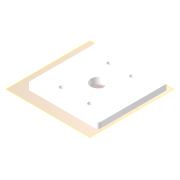
# Autodesk Inventor part: 20_Cube_Adapter_Zstage_manual
Saved by Autodesk Inventor 2022 (Build 260153000, 153)
## iProperties
Created: 2017-06-20
Part Number: 20_Cube_Adapter_Zstage_manual
Material: Generisch
Document SubType Name: Modeling
Designer: diederichbenedict
Density: 1 g/cm^3
Appearance: Weiß
Mass: 5.4697 g
Surface Area: 48.9743 cm^2
Volume: 5.4697 cm^3
Catalog Web Link: isInjectionmolded
Vendor: openUC2
d_part: 50,000 mm
d_o: 40,000 mm
d_i: 40,000 mm
Author: diederichbenedict
Autodesk Inventor part; units mm, degrees
ref_plane "YZ Plane" through (0, 0, 0) normal (1, 0, 0) x (0, 1, 0)
ref_plane "XZ Plane" through (0, 0, 0) normal (0, 1, 0) x (-1, 0, 0)
ref_plane "XY Plane" through (0, 0, 0) normal (0, 0, 1) x (1, 0, 0)
ref_plane "Arbeitsebene15" through (-38.58009, 58.540516, -23.010083) normal (0, 0, 1) x (1, 0, 0)
sketch "Skizze38" plane through (-38.58009, 58.540516, -23.010083) normal (0, 0, 1) x (1, 0, 0)
  circle A0 centre (27, 33.3) radius 3
  circle A1 centre (-8.3, 27) radius 3
  circle A2 centre (-2, -8.3) radius 3
  circle A3 centre (33.3, -2) radius 3
  circle A4 centre (27, -8.3) radius 3
  circle A5 centre (-8.3, -2) radius 3
  circle A6 centre (-2, 33.3) radius 3
  circle A7 centre (33.3, 27) radius 3
  line L0 (27.5, 29.5) -> (-2.5, 29.5)
  arc A8 (29.5, 27.5) -> (27.5, 29.5) centre (27.5, 27.5) ccw
  line L1 (29.5, 27.5) -> (29.5, -2.5)
  arc A9 (27.5, -4.5) -> (29.5, -2.5) centre (27.5, -2.5) ccw
  line L2 (-2.5, -4.5) -> (27.5, -4.5)
  arc A10 (-4.5, -2.5) -> (-2.5, -4.5) centre (-2.5, -2.5) ccw
  line L3 (-4.5, -2.5) -> (-4.5, 27.5)
  arc A11 (-2.5, 29.5) -> (-4.5, 27.5) centre (-2.5, 27.5) ccw
  circle A12 centre (33.5, 33.5) radius 2.5
  circle A13 centre (-8.5, -8.5) radius 2.5
  circle A14 centre (33.5, -8.5) radius 2.5
  circle A15 centre (-8.5, 33.5) radius 2.5
  line L4 (-11.75, -10.5) -> (-11.75, 8.25)
  arc A16 (-11.75, -10.5) -> (-10.5, -11.75) centre (-10.5, -10.5) ccw
  line L5 (8.25, -11.75) -> (-10.5, -11.75)
  line L6 (8.25, -13.877389) -> (8.25, -11.75)
  arc A17 (7.405556, -14.865216) -> (8.25, -13.877389) centre (7.25, -13.877389) ccw
  arc A18 (7.405556, -14.865216) -> (7.6, -17.35) centre (7.6, -16.1) ccw
  line L7 (17.4, -17.35) -> (7.6, -17.35)
  arc A19 (17.4, -17.35) -> (17.594444, -14.865216) centre (17.4, -16.1) ccw
  arc A20 (16.75, -13.877389) -> (17.594444, -14.865216) centre (17.75, -13.877389) ccw
  line L8 (16.75, -11.75) -> (16.75, -13.877389)
  line L9 (35.5, -11.75) -> (16.75, -11.75)
  arc A21 (35.5, -11.75) -> (36.75, -10.5) centre (35.5, -10.5) ccw
  line L10 (36.75, 6.487451) -> (36.75, -10.5)
  arc A22 (36.75, 6.487451) -> (36.55605, 6.521706) centre (36.65, 6.487451) ccw
  arc A23 (31.3, 7.45) -> (36.55605, 6.521706) centre (34.01, 7.45) ccw
  line L11 (31.3, 17.55) -> (31.3, 7.45)
  arc A24 (36.55605, 18.478294) -> (31.3, 17.55) centre (34.01, 17.55) ccw
  arc A25 (36.55605, 18.478294) -> (36.75, 18.512549) centre (36.65, 18.512549) ccw
  line L12 (36.75, 35.5) -> (36.75, 18.512549)
  arc A26 (36.75, 35.5) -> (35.5, 36.75) centre (35.5, 35.5) ccw
  line L13 (18.512549, 36.75) -> (35.5, 36.75)
  arc A27 (18.512549, 36.75) -> (18.478294, 36.55605) centre (18.512549, 36.65) ccw
  arc A28 (17.55, 31.3) -> (18.478294, 36.55605) centre (17.55, 34.01) ccw
  line L14 (7.45, 31.3) -> (17.55, 31.3)
  arc A29 (6.521706, 36.55605) -> (7.45, 31.3) centre (7.45, 34.01) ccw
  arc A30 (6.521706, 36.55605) -> (6.487451, 36.75) centre (6.487451, 36.65) ccw
  line L15 (-10.5, 36.75) -> (6.487451, 36.75)
  arc A31 (-10.5, 36.75) -> (-11.75, 35.5) centre (-10.5, 35.5) ccw
  line L16 (-11.75, 16.75) -> (-11.75, 35.5)
  line L17 (-13.877389, 16.75) -> (-11.75, 16.75)
  arc A32 (-14.865216, 17.594444) -> (-13.877389, 16.75) centre (-13.877389, 17.75) ccw
  arc A33 (-14.865216, 17.594444) -> (-17.35, 17.4) centre (-16.1, 17.4) ccw
  line L18 (-17.35, 7.6) -> (-17.35, 17.4)
  arc A34 (-17.35, 7.6) -> (-14.865216, 7.405556) centre (-16.1, 7.6) ccw
  arc A35 (-13.877389, 8.25) -> (-14.865216, 7.405556) centre (-13.877389, 7.25) ccw
  line L19 (-11.75, 8.25) -> (-13.877389, 8.25)
  line L20 (-2.5, 30.1) -> (27.5, 30.1)
  arc A36 (30.1, 27.5) -> (27.5, 30.1) centre (27.5, 27.5) ccw
  line L21 (30.1, 27.5) -> (30.1, -2.5)
  arc A37 (27.5, -5.1) -> (30.1, -2.5) centre (27.5, -2.5) ccw
  line L22 (27.5, -5.1) -> (-2.5, -5.1)
  arc A38 (-5.1, -2.5) -> (-2.5, -5.1) centre (-2.5, -2.5) ccw
  line L23 (-5.1, -2.5) -> (-5.1, 27.5)
  arc A39 (-2.5, 30.1) -> (-5.1, 27.5) centre (-2.5, 27.5) ccw
  point P0 (38.58009, -58.540516)
  dimension "d425" = 0.6
  constraints: 8 end point, 8 point on circle, 4 centre point, 7 other
  measures "d425" distance between parallel lines of L0 L20
sketch "Skizze38 outline for Extrusion20" plane through (-38.58009, 58.540516, -23.010083) normal (0, 0, 1) x (1, 0, 0)
  arc A0 (-5.1, -2.5) -> (-2.5, -5.1) centre (-2.5, -2.5) ccw
  line L0 (-5.1, 27.5) -> (-5.1, -2.5)
  arc A1 (-2.5, 30.1) -> (-5.1, 27.5) centre (-2.5, 27.5) ccw
  line L1 (27.5, 30.1) -> (-2.5, 30.1)
  arc A2 (30.1, 27.5) -> (27.5, 30.1) centre (27.5, 27.5) ccw
  line L2 (30.1, -2.5) -> (30.1, 27.5)
  arc A3 (27.5, -5.1) -> (30.1, -2.5) centre (27.5, -2.5) ccw
  line L3 (-2.5, -5.1) -> (27.5, -5.1)
extrude "Extrusion20" add sketch "Skizze38 outline for Extrusion20" against normal blind 5 draft -3
sketch "Skizze39" plane through (-38.58009, 58.540516, -23.010083) normal (0, 0, 1) x (1, 0, 0)
  line L0 (-2.5, -5.1) -> (27.5, -5.1) projected
  arc A0 (27.5, -5.1) -> (30.1, -2.5) centre (27.5, -2.5) ccw projected
  line L1 (30.1, -2.5) -> (30.1, 27.5) projected
  arc A1 (30.1, 27.5) -> (27.5, 30.1) centre (27.5, 27.5) ccw projected
  line L2 (27.5, 30.1) -> (-2.5, 30.1) projected
  arc A2 (-2.5, 30.1) -> (-5.1, 27.5) centre (-2.5, 27.5) ccw projected
  line L3 (-5.1, 27.5) -> (-5.1, -2.5) projected
  arc A3 (-5.1, -2.5) -> (-2.5, -5.1) centre (-2.5, -2.5) ccw projected
  line L4 (17.5, -12.5) -> (35.5, -12.5) projected
  line L5 (-10.5, 37.5) -> (35.5, 37.5)
  line L6 (37.5, 35.5) -> (37.5, -10.5)
  line L7 (35.5, -12.5) -> (-10.5, -12.5)
  line L8 (-12.5, -10.5) -> (-12.5, 35.5)
  line L9 (-12.5, 37.5) -> (37.5, -12.5) construction
  line L10 (37.5, 37.5) -> (-12.5, -12.5) construction
  arc A4 (37.5, 35.5) -> (35.5, 37.5) centre (35.5, 35.5) ccw projected
  arc A5 (37.5, 35.5) -> (35.5, 37.5) centre (35.5, 35.5) ccw
  arc A6 (-10.5, 37.5) -> (-12.5, 35.5) centre (-10.5, 35.5) ccw
  arc A7 (-12.5, -10.5) -> (-10.5, -12.5) centre (-10.5, -10.5) ccw
  arc A8 (35.5, -12.5) -> (37.5, -10.5) centre (35.5, -10.5) ccw
  point P0 (38.58009, -58.540516)
  point P1 (12.5, 12.5)
  point P2 (35.5, -12.5)
  dimension "d428" = 50
  dimension "d429" = 50
  dimension "d430" = 2
  constraints: 12 end point, 8 point on circle, 8 point on line, 8 tangent, 4 centre point, 3 equal radius, 2 midpoint, 2 parallel, 1 horizontal, 1 perpendicular
  measures "d428" distance of L9.end L10.end
  measures "d429" distance of L10.start L9.end
  measures "d430" radius of A5
extrude "Extrusion21" add sketch "Skizze39" along normal blind 4 contours A3 L3 A2 L2 A1 L1 A0 L0 | L7 A7 L8 A6 L5 A4 L6 A8 L4
sketch "Skizze40" plane through (-38.58009, 58.540516, -19.010083) normal (0, 0, 1) x (1, 0, 0)
  arc A0 (-10.5, 37.5) -> (-12.5, 35.5) centre (-10.5, 35.5) ccw projected
  line L0 (-12.5, 35.5) -> (-12.5, -10.5) projected
  arc A1 (-12.5, -10.5) -> (-10.5, -12.5) centre (-10.5, -10.5) ccw projected
  line L1 (-10.5, -12.5) -> (35.5, -12.5) projected
  arc A2 (35.5, -12.5) -> (37.5, -10.5) centre (35.5, -10.5) ccw projected
  line L2 (37.5, -10.5) -> (37.5, 35.5) projected
  arc A3 (37.5, 35.5) -> (35.5, 37.5) centre (35.5, 35.5) ccw projected
  line L3 (35.5, 37.5) -> (-10.5, 37.5) projected
  circle A4 centre (12.5, 12.5) radius 5
  line L4 (-2.5, 20) -> (27.5, 20) construction
  line L5 (27.5, 20) -> (27.5, -8) construction
  line L6 (27.5, -8) -> (-2.5, -8) construction
  line L7 (-2.5, -8) -> (-2.5, 20) construction
  circle A5 centre (2.5, -3.1) radius 1.5
  circle A6 centre (22.5, -3.1) radius 1.5
  point P0 (38.58009, -58.540516)
  dimension "d433" = 10
  dimension "d434" = 30
  dimension "d435" = 28
  dimension "d436" = 15
  dimension "d437" = 25
  dimension "d438" = 25
  dimension "d439" = 7.5
  dimension "d440" = 3
  dimension "d441" = 3
  dimension "d442" = 5
  dimension "d443" = 5
  dimension "d466" = 15.6
  dimension "d467" = 15.6
  constraints: 8 end point, 3 centre point, 2 parallel, 1 horizontal, 1 perpendicular
  measures "d433" diameter of A4
  measures "d434" distance of L5.end L6.end
  measures "d435" distance of L4.end L5.end
  measures "d436" distance from line of A4.centre L7
  measures "d437" distance from line of A4.centre L0
  measures "d438" distance from line of L3 A4.centre
  measures "d439" distance from line of A4.centre L4
  measures "d440" diameter of A5
  measures "d441" diameter of A6
  measures "d442" distance from line of A5.centre L7
  measures "d443" distance from line of L5 A6.centre
  measures "d466" vertical distance of A4.centre A6.centre
  measures "d467" vertical distance of A4.centre A5.centre
extrude "Extrusion22" cut sketch "Skizze40" against normal through all contours A4 | A5 | A6
sketch "Skizze41" plane through (-38.58009, 58.540516, -28.010083) normal (0, 0, -1) x (-1, 0, 0)
  circle A0 centre (-12.5, 12.5) radius 5 projected
  circle A1 centre (-4.5, 28.5) radius 1.4
  circle A2 centre (-20.5, 28.5) radius 1.4
  circle A3 centre (-2.5, -3.1) radius 1.5 projected
  circle A4 centre (-22.5, -3.1) radius 1.5 projected
  point P0 (-38.58009, -58.540516)
  point P1 (-3.17813, -4.837961)
  point P2 (-1.82187, -4.837961)
  point P3 (-23.17813, -4.837961)
  point P4 (-21.82187, -4.837961)
  dimension "d456" = 2.8
  dimension "d457" = 2.8
  dimension "d458" = 16
  dimension "d459" = 16
  dimension "d460" = 8
  dimension "d461" = 8
  constraints: 2 centre point, 2 other
  measures "d456" diameter of A1
  measures "d457" diameter of A2
  measures "d458" vertical distance of A2.centre A0.centre
  measures "d459" vertical distance of A0.centre A1.centre
  measures "d460" horizontal distance of A1.centre A0.centre
  measures "d461" horizontal distance of A0.centre A2.centre
hole "Bohrung10" at (-34.08009, 87.040516, -28.010083) at (-18.08009, 87.040516, -28.010083) at (-36.08009, 55.440516, -28.010083) at (-16.08009, 55.440516, -28.010083) direction (0, 0, 1) diameter 2.8 end through all counterbore diameter 6.5 counterbore depth 8
ref_plane "Arbeitsebene16" through (-38.58009, 58.540516, -24.010083) normal (0, 0, -1) x (-1, 0, 0)
sketch "Skizze44" plane through (-38.58009, 58.540516, -24.010083) normal (0, 0, -1) x (-1, 0, 0)
  circle A0 centre (-12.5, 12.5) radius 5 projected
  circle A1 centre (-12.5, 12.5) radius 16
  point P0 (-38.58009, -58.540516)
  dimension "d472" = 32
  constraints: 1 centre point, 1 coincident
  measures "d472" diameter of A1
extrude "Extrusion25" cut sketch "Skizze44" along normal through all draft 5 contours A0 | A1
equation "\"d_i\" = 40"
equation "\"d_o\" = 40"
equation "\"d_part\" = 50"
equation "\"d6\" = 0"
equation "\"d7\" = 0"
equation "\"d8\" = 0"
equation "\"d9\" = 0"
equation "\"d13\" = 0"
equation "\"d14\" = 0"
equation "\"d20\" = 0"
equation "\"d21\" = 0"
equation "\"d22\" = 0"
equation "\"d23\" = 0"
equation "\"d24\" = 0"
equation "\"d25\" = 3"
equation "\"d26\" = 0"
equation "\"d27\" = 0"
equation "\"d28\" = 0"
equation "\"d29\" = 0"
equation "\"d30\" = 0"
equation "\"d31\" = 0"
equation "\"d32\" = 0"
equation "\"d33\" = 0"
equation "\"d34\" = 0"
equation "\"d46\" = 0"
equation "\"d47\" = 0"
equation "\"d48\" = 0"
equation "\"d50\" = 0"
equation "\"d51\" = 0"
equation "\"d52\" = 0"
equation "\"d53\" = 0"
equation "\"d54\" = 0"
equation "\"d55\" = 0"
equation "\"d56\" = 0"
equation "\"d57\" = 0"
equation "\"d58\" = 0"
equation "\"d59\" = 0"
equation "\"magnet_offset\" = 0"
equation "\"screw_offset\" = 0"
equation "\"mal_puzzle_offset\" = 0"
equation "\"fem_puzzle_offset\" = 0"
